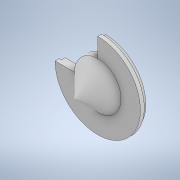
# Autodesk Inventor part: крышка кожуха пушки
Saved by Autodesk Inventor 2020.1 (Build 241239000, 239)
## iProperties
Created: 2022-04-02
Part Number: крышка кожуха пушки
Material: Типовые
Document SubType Name: Modeling
Designer: User
Density: 1 g/cm^3
Appearance: По умолчанию
Author: User
Autodesk Inventor part; units mm, degrees
ref_plane "YZ Plane" through (0, 0, 0) normal (1, 0, 0) x (0, 1, 0)
ref_plane "XZ Plane" through (0, 0, 0) normal (0, 1, 0) x (-1, 0, 0)
ref_plane "XY Plane" through (0, 0, 0) normal (0, 0, 1) x (1, 0, 0)
sketch "Эскиз1" plane through (0, 0, 0) normal (0, 0, 1) x (1, 0, 0)
  circle A0 centre (0, 0) radius 7.5
  circle A1 centre (0, 0) radius 20
  circle A2 centre (0, 0) radius 22
  line L0 (0, 0) -> (-22, 0)
  line L1 (0, 0) -> (0, 22)
  line L2 (-22, 0) -> (-20, 0)
  line L3 (-20, 0) -> (-20, -4)
  line L4 (-20, -4) -> (-22, -4)
  line L5 (-22, -4) -> (-22, 0)
  point P0 (20, 0)
  point P1 (22, 0)
  point P2 (0, 20)
  point P3 (-20, 0)
  point P4 (-21.6333, -4)
  dimension "d1" = 40
  dimension "d0" = 15
  dimension "d2" = 2
  dimension "d10" = 4
  constraints: 12 end point, 3 coincident, 3 point on circle, 2 centre point, 2 horizontal, 2 parallel, 2 perpendicular, 3 other
  measures "d0" diameter of A0
  measures "d2" distance of A2.start point (20, 0)
  measures "d10" distance of L4.end L0.end
extrude "Выдавливание1" add sketch "Эскиз1" along normal blind 215 contours L1 A2 L4 L3 A1 | L3 L4 A2 L0
sketch "Эскиз2" plane through (0, 0, 215) normal (0, 0, 1) x (1, 0, 0)
  arc A0 (-20, 0) -> (0, 20) centre (0, 0) ccw projected
  arc A1 (-22, 0) -> (0, 22) centre (0, 0) ccw projected
  arc A2 (-22, 0) -> (0, 22) centre (0, 0) ccw projected
  line L0 (0, 22) -> (0, 20) projected
  arc A3 (-20, 0) -> (0, 20) centre (0, 0) ccw projected
  line L1 (-20, 0) -> (-22, 0) projected
  circle A4 centre (0, 0) radius 8
  line L2 (0, 8) -> (0, 20)
  line L3 (-8, 0) -> (-20.5, 0)
  circle A5 centre (0, 0) radius 12
  point P0 (0, 20)
  point P1 (-12, 0)
  point P2 (0, 12)
  dimension "d5" = 16
  dimension "d15" = 4
  constraints: 4 end point, 2 coincident, 2 point on circle, 1 centre point, 1 point on line, 1 vertical, 3 other
  measures "d5" diameter of A4
  measures "d15" distance of point (-12, 0) L3.start
extrude "Выдавливание2" add sketch "Эскиз2" against normal blind 4 contours L3 A5 L2 A0 | A5 L2 A4 L3 | L3 A4 L2 A5
sketch "Эскиз3" plane through (0, 0, 0) normal (0, 0, -1) x (-1, 0, 0)
  line L0 (20, 0) -> (12, 0) projected
  circle A0 centre (0, 0) radius 8 projected
  line L1 (0, 12) -> (0, 20) projected
  arc A1 (0, 20) -> (20, 0) centre (0, 0) ccw projected
  arc A2 (12, 0) -> (0, 12) centre (0, 0) ccw projected
extrude "Выдавливание3" add sketch "Эскиз3" against normal blind 4
sketch "Эскиз4" plane through (0, 0, 0) normal (0, 0, -1) x (-1, 0, 0)
  arc A0 (0, 20) -> (20, 0) centre (0, 0) ccw projected
  line L0 (20, 0) -> (60, 0)
  line L1 (60, 0) -> (60, -4)
  line L2 (60, -4) -> (20, -4)
  line L3 (20, -4) -> (20, 0)
  dimension "d11" = 40
  dimension "d12" = 4
  constraints: 8 end point, 2 parallel, 1 horizontal, 1 perpendicular
  measures "d11" distance of L1.end L2.end
  measures "d12" distance of L0.end L1.end
extrude "Выдавливание4" add sketch "Эскиз4" against normal blind 60
sketch "Эскиз5" plane through (-60, -4, 0) normal (0, -1, 0) x (1, 0, 0)
  line L0 (10, 50) -> (25, 50)
  line L1 (25, 50) -> (25, 45)
  line L2 (25, 45) -> (10, 45)
  line L3 (10, 45) -> (10, 50)
  line L4 (10, 15) -> (25, 15)
  line L5 (25, 15) -> (25, 10)
  line L6 (25, 10) -> (10, 10)
  line L7 (10, 10) -> (10, 15)
  line L8 (38.3667, 0) -> (0, 0) projected
  line L9 (0, 0) -> (0, 60) projected
  line L10 (0, 30) -> (39.4889, 30)
  line L11 (38.3667, 60) -> (38.3667, 0) projected
  line L12 (10, 27.5) -> (25, 27.5)
  line L13 (25, 27.5) -> (25, 32.5)
  line L14 (25, 32.5) -> (10, 32.5)
  line L15 (10, 32.5) -> (10, 27.5)
  point P0 (60, 0)
  dimension "d16" = 10
  dimension "d17" = 10
  dimension "d19" = 5
  dimension "d22" = 15
  dimension "d23" = 0
  constraints: 26 end point, 6 parallel, 4 equal length, 4 horizontal, 3 perpendicular, 1 midpoint, 4 other
  measures "d16" distance from line of L8 L6.end
  measures "d17" distance from line of L9 L6.end
  measures "d19" distance of L6.end L4.start
  measures "d22" distance of L5.end L6.end
  measures "d23" horizontal distance of L4.start L12.start
extrude "Выдавливание5" cut sketch "Эскиз5" against normal blind 10 contours L0 L1 L2 L3 | L4 L5 L6 L7 | L13 L12 L15 L10 | L10 L15 L14 L13
sketch "Эскиз6" plane through (-60, -4, 0) normal (-1, 0, 0) x (0, 0, 1)
  line L0 (211, 32.0308) -> (-1.8272, 32.0308)
  line L1 (-1.8272, 32.0308) -> (-1.8272, -28.2031)
  line L2 (-1.8272, -28.2031) -> (211, -28.2031)
  line L3 (211, -28.2031) -> (211, 32.0308)
  point P0 (0, 4)
  constraints: 8 end point, 2 parallel, 1 horizontal, 1 perpendicular
extrude "Выдавливание6" cut sketch "Эскиз6" against normal blind 100
sketch "Эскиз7" plane through (0, 0, 211) normal (0, 0, -1) x (-1, 0, 0)
  arc A0 (0, 22) -> (22, 0) centre (0, 0) ccw projected
  circle A1 centre (0, 0) radius 22
  circle A2 centre (0, 0) radius 20.8
  point P0 (0, 20.8)
  point P1 (22, 0)
  dimension "d26" = 1.2
  constraints: 2 coincident, 1 vertical alignment, 5 other
  measures "d26" distance of A0.start point (0, 20.8)
extrude "Выдавливание7" cut sketch "Эскиз7" against normal blind 2
sketch "Эскиз9" plane through (0, 0, 0) normal (0, 1, 0) x (-1, 0, 0)
  line L0 (12, 215) -> (0, 215) projected
  circle A0 centre (0, 215) radius 12
  line L1 (0, 215) -> (0, 227)
  line L2 (12, 215) -> (0, 227)
  point P0 (0, 0)
  constraints: 4 end point, 3 point on circle, 1 centre point, 1 vertical
revolve "Вращение1" add sketch "Эскиз9" angle 360 about axis through (0, 0, 215) along (0, 0, 1) contours L0 L1 L2
sketch "Эскиз10" plane through (0, 0, 215) normal (0, 0, -1) x (-1, 0, 0)
  circle A0 centre (0, 0) radius 3
  dimension "d30" = 6
  constraints: 1 centre point, 1 coincident
  measures "d30" diameter of A0
extrude "Выдавливание8" cut sketch "Эскиз10" against normal blind 5
